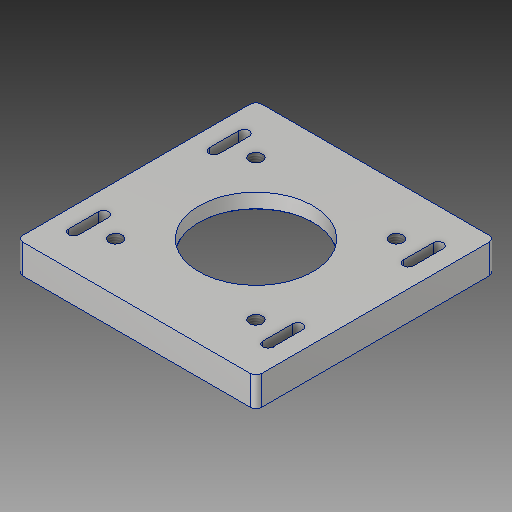
# Autodesk Inventor part: Z-Motoraufnahme
Saved by Autodesk Inventor 2019 (Build 230136000, 136)
## iProperties
Created: 2021-04-24
Part Number: Z-Motoraufnahme
Material: Aluminium 6061
Document SubType Name: Modeling
Designer: Michael Sumper
Density: 2.7 g/cm^3
Appearance: Aluminium - flach
Mass: 103.162 g
Surface Area: 163.877 cm^2
Volume: 38.208 cm^3
Author: Michael Sumper
Autodesk Inventor part; units mm, degrees
ref_plane "YZ Plane" through (0, 0, 0) normal (1, 0, 0) x (0, 1, 0)
ref_plane "XZ Plane" through (0, 0, 0) normal (0, 1, 0) x (-1, 0, 0)
ref_plane "XY Plane" through (0, 0, 0) normal (0, 0, 1) x (1, 0, 0)
sketch "Skizze1" plane through (0, 0, 0) normal (0, 1, 0) x (-1, 0, 0)
  circle A0 centre (0, 0) radius 19.1
  line L0 (-23.5, 23.5) -> (23.5, 23.5) construction
  line L1 (23.5, 23.5) -> (23.5, -23.5) construction
  line L2 (23.5, -23.5) -> (-23.5, -23.5) construction
  line L3 (-23.5, -23.5) -> (-23.5, 23.5) construction
  line L4 (-23.5, 23.5) -> (23.5, -23.5) construction
  line L5 (23.5, 23.5) -> (-23.5, -23.5) construction
  circle A1 centre (23.5, -23.5) radius 2.2
  circle A2 centre (23.5, 23.5) radius 2.2
  circle A3 centre (-23.5, 23.5) radius 2.2
  circle A4 centre (-23.5, -23.5) radius 2.2
  line L6 (-40, 40) -> (40, 40)
  line L7 (40, 40) -> (40, -40)
  line L8 (40, -40) -> (-40, -40)
  line L9 (-40, -40) -> (-40, 40)
  line L10 (-40, 40) -> (40, -40) construction
  line L11 (40, 40) -> (-40, -40) construction
  line L12 (-32.5, 23.5) -> (32.5, 23.5) construction
  line L13 (32.5, 23.5) -> (32.5, -23.5) construction
  line L14 (32.5, -23.5) -> (-32.5, -23.5) construction
  line L15 (-32.5, -23.5) -> (-32.5, 23.5) construction
  line L16 (-32.5, 23.5) -> (32.5, -23.5) construction
  line L17 (32.5, 23.5) -> (-32.5, -23.5) construction
  line L18 (32.5, -18.5) -> (32.5, -28.5) construction
  line L19 (30.8, -18.5) -> (30.8, -28.5)
  line L20 (34.2, -28.5) -> (34.2, -18.5)
  arc A5 (34.2, -18.5) -> (30.8, -18.5) centre (32.5, -18.5) ccw
  arc A6 (30.8, -28.5) -> (34.2, -28.5) centre (32.5, -28.5) ccw
  line L21 (32.5, 28.5) -> (32.5, 18.5) construction
  line L22 (30.8, 28.5) -> (30.8, 18.5)
  line L23 (34.2, 18.5) -> (34.2, 28.5)
  arc A7 (34.2, 28.5) -> (30.8, 28.5) centre (32.5, 28.5) ccw
  arc A8 (30.8, 18.5) -> (34.2, 18.5) centre (32.5, 18.5) ccw
  line L24 (-32.5, 28.5) -> (-32.5, 18.5) construction
  line L25 (-34.2, 28.5) -> (-34.2, 18.5)
  line L26 (-30.8, 18.5) -> (-30.8, 28.5)
  arc A9 (-30.8, 28.5) -> (-34.2, 28.5) centre (-32.5, 28.5) ccw
  arc A10 (-34.2, 18.5) -> (-30.8, 18.5) centre (-32.5, 18.5) ccw
  line L27 (-32.5, -18.5) -> (-32.5, -28.5) construction
  line L28 (-34.2, -18.5) -> (-34.2, -28.5)
  line L29 (-30.8, -28.5) -> (-30.8, -18.5)
  arc A11 (-30.8, -18.5) -> (-34.2, -18.5) centre (-32.5, -18.5) ccw
  arc A12 (-34.2, -28.5) -> (-30.8, -28.5) centre (-32.5, -28.5) ccw
  line L30 (-30, 30) -> (30, 30)
  line L31 (30, 30) -> (30, -30)
  line L32 (30, -30) -> (-30, -30)
  line L33 (-30, -30) -> (-30, 30)
  line L34 (-30, 30) -> (30, -30) construction
  line L35 (30, 30) -> (-30, -30) construction
  dimension "d31" = 38.2
  dimension "d32" = 47
  dimension "d33" = 47
  dimension "d34" = 4.4
  dimension "d35" = 4.4
  dimension "d36" = 4.4
  dimension "d37" = 4.4
  dimension "d38" = 80
  dimension "d39" = 80
  dimension "d40" = 65
  dimension "d41" = 47
  dimension "d42" = 5
  dimension "d43" = 3.4
  dimension "d44" = 5
  dimension "d45" = 3.4
  dimension "d46" = 5
  dimension "d47" = 3.4
  dimension "d48" = 5
  dimension "d49" = 3.4
  dimension "d50" = 60
  dimension "d51" = 60
  constraints: 80 end point, 16 point on circle, 16 tangent, 13 centre point, 12 midpoint, 12 parallel, 5 coincident, 5 perpendicular, 4 horizontal, 3 point on line
  measures "d31" diameter of A0
  measures "d32" distance of L1.end L2.end
  measures "d33" distance of L0.end L1.end
  measures "d34" diameter of A1
  measures "d35" diameter of A2
  measures "d36" diameter of A3
  measures "d37" diameter of A4
  measures "d38" distance of L7.end L8.end
  measures "d39" distance of L6.end L7.end
  measures "d40" distance of L13.end L14.end
  measures "d41" distance of L12.end L13.end
  measures "d42" distance of L13.end L18.end
  measures "d43" diameter of A6
  measures "d44" distance of L12.end L21.end
  measures "d45" diameter of A8
  measures "d46" distance of L12.start L24.end
  measures "d47" diameter of A10
  measures "d48" distance of L14.end L27.end
  measures "d49" diameter of A12
  measures "d50" distance of L31.end L32.end
  measures "d51" distance of L30.end L31.end
extrude "Extrusion1" add sketch "Skizze1" against normal blind 10 contours L6 L7 L8 L9
extrude "Extrusion2" add sketch "Skizze1" against normal blind 5 contours L30 L31 L32 L33
fillet "Rundung1" radius 2 8 edges at (-40, -5, 40) (40, -5, -40) (-40, -5, -40) (40, -5, 40) (30, -7.5, 30) (-30, -7.5, -30) (30, -7.5, -30) (-30, -7.5, 30)
chamfer "Fase1" distance 0.2 angle 45 37 edges at (25.7, -5, 23.5) (30, -10, 0) (29.4142, -10, -29.4142) (0, -10, -30) (-29.4142, -10, -29.4142) (-30, -10, 0) (-29.4142, -10, 29.4142) (0, -10, 30) (29.4142, -10, 29.4142) (32.5, -10, 16.8) (30.8, -10, 23.5) (32.5, -10, 30.2) (34.2, -10, 23.5) (19.1, -5, 0) (25.7, -5, -23.5) (-21.3, -5, -23.5) (-21.3, -5, 23.5) (-32.5, -10, 16.8) (-34.2, -10, 23.5) (-32.5, -10, 30.2) (-30.8, -10, 23.5) (-32.5, -10, -16.8) (-30.8, -10, -23.5) (-32.5, -10, -30.2) (-34.2, -10, -23.5) (0, -10, -40) (39.4142, -10, -39.4142) (40, -10, 0) (39.4142, -10, 39.4142) (0, -10, 40) (-39.4142, -10, 39.4142) (-40, -10, 0) (-39.4142, -10, -39.4142) (32.5, -10, -16.8) (34.2, -10, -23.5) (32.5, -10, -30.2) (30.8, -10, -23.5)
thread "Gewinde1" size "M5x0.8" class "6H" standard "ANSI Metric M Profile" full length
thread "Gewinde2" size "M5x0.8" class "6H" standard "ANSI Metric M Profile" full length
thread "Gewinde3" size "M5x0.8" class "6H" standard "ANSI Metric M Profile" full length
thread "Gewinde4" size "M5x0.8" class "6H" standard "ANSI Metric M Profile" full length
